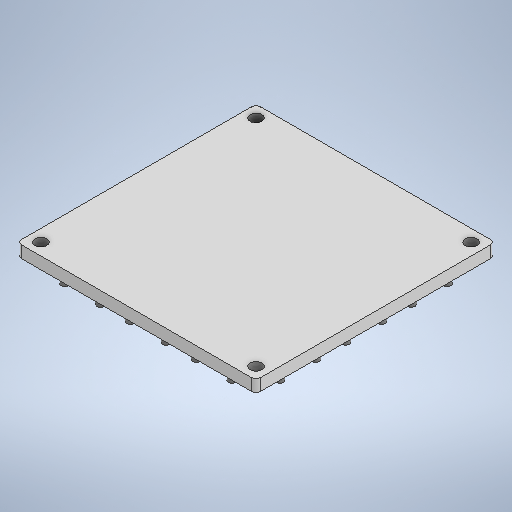
# Autodesk Inventor part: plateau
Saved by Autodesk Inventor 2025 (Build 290162010, 162A)
## iProperties
Created: 2025-02-16
Part Number: plateau
Material: Générique
Document SubType Name: Modeling
Designer: arthu
Density: 1 g/cm^3
Appearance: Par défaut
Author: arthu
Autodesk Inventor part; units mm, degrees
ref_plane "YZ Plane" through (0, 0, 0) normal (1, 0, 0) x (0, 1, 0)
ref_plane "XZ Plane" through (0, 0, 0) normal (0, 1, 0) x (-1, 0, 0)
ref_plane "XY Plane" through (0, 0, 0) normal (0, 0, 1) x (1, 0, 0)
sketch "Esquisse1" plane through (0, 0, 0) normal (0, 1, 0) x (-1, 0, 0)
  line L0 (0, 0) -> (100, 0)
  line L1 (100, 0) -> (100, -100)
  line L2 (100, -100) -> (0, -100)
  line L3 (0, -100) -> (0, 0)
  dimension "d0" = 100
  dimension "d1" = 100
  constraints: 8 end point, 2 parallel, 1 horizontal, 1 perpendicular
  measures "d0" distance of L1.end L2.end
  measures "d1" distance of L0.end L1.end
extrude "Extrusion1" add sketch "Esquisse1" along normal blind 5
sketch "Esquisse3" plane through (0, 0, 0) normal (0, -1, 0) x (1, 0, 0)
  line L0 (0, -100) -> (-100, -100) projected
  line L1 (0, -100) -> (-4.9999, -95)
  circle A0 centre (-4.9999, -95) radius 1.6952
  point P0 (0, 0)
  dimension "d4" = 7.071
  constraints: 2 end point, 1 centre point, 1 coincident
  measures "d4" distance of L0.start L1.end
hole "Perçage1" at (-4.9999, 0, -95) direction (0, 1, 0) diameter 4.9587 depth 5 thread size "M5.5x0.5" class "6H" standard "ISO Metric profile"
pattern_linear "Réseau rectangulaire1" count 2 spacing 90 along (0, 0, 1) count 2 spacing 90 along (-1, 0, 0) of "Perçage1"
fillet "Congé1" radius 2 4 edges at (0, 2.5, 0) (-100, 2.5, 0) (-100, 2.5, -100) (0, 2.5, -100)
sketch "Esquisse7" plane through (0, 0, 0) normal (0, -1, 0) x (1, 0, 0)
  circle A0 centre (-4.9999, -5) radius 2.4794 projected
  circle A1 centre (-94.9999, -95) radius 2.4794 projected
  line L0 (-4.9999, -5) -> (-94.9999, -5)
  line L1 (-94.9999, -5) -> (-94.9999, -95)
  line L2 (-94.9999, -95) -> (-4.9999, -95)
  line L3 (-4.9999, -95) -> (-4.9999, -5)
  line L4 (-49.9999, -5) -> (-49.9999, -95)
  line L5 (-4.9999, -50) -> (-94.9999, -50)
  line L6 (-49.9999, -95) -> (-42.4999, -95)
  line L7 (-49.9999, -95) -> (-57.4999, -95)
  circle A2 centre (-57.4999, -95) radius 1.55
  circle A3 centre (-42.4999, -95) radius 1.55
  line L8 (-94.9999, -95) -> (-84.9999, -95)
  line L9 (-84.9999, -95) -> (-69.9999, -95)
  circle A4 centre (-69.9999, -95) radius 1.55
  circle A5 centre (-84.9999, -95) radius 1.55
  circle A6 centre (-4.9999, -95) radius 2.4794 projected
  line L10 (-4.9999, -95) -> (-14.9999, -95)
  line L11 (-14.9999, -95) -> (-29.9999, -95)
  circle A7 centre (-14.9999, -95) radius 1.55
  circle A8 centre (-29.9999, -95) radius 1.55
  circle A9 centre (-14.9999, -5) radius 1.55
  circle A10 centre (-29.9999, -5) radius 1.55
  circle A11 centre (-42.4999, -5) radius 1.55
  circle A12 centre (-57.4999, -5) radius 1.55
  circle A13 centre (-69.9999, -5) radius 1.55
  circle A14 centre (-84.9999, -5) radius 1.55
  circle A15 centre (-4.9999, -85) radius 1.55
  circle A16 centre (-4.9999, -70) radius 1.55
  circle A17 centre (-4.9999, -57.5) radius 1.55
  circle A18 centre (-4.9999, -42.5) radius 1.55
  circle A19 centre (-4.9999, -30) radius 1.55
  circle A20 centre (-4.9999, -15) radius 1.55
  circle A21 centre (-94.9999, -15) radius 1.55
  circle A22 centre (-94.9999, -30) radius 1.55
  circle A23 centre (-94.9999, -42.5) radius 1.55
  circle A24 centre (-94.9999, -57.5) radius 1.55
  circle A25 centre (-94.9999, -70) radius 1.55
  circle A26 centre (-94.9999, -85) radius 1.55
  point P0 (0, 0)
  dimension "d35" = 7.5
  dimension "d36" = 7.5
  dimension "d37" = 3.1
  dimension "d38" = 3.1
  dimension "d39" = 10
  dimension "d40" = 15
  dimension "d41" = 3.1
  dimension "d42" = 3.1
  dimension "d43" = 10
  dimension "d44" = 15
  dimension "d45" = 3.1
  dimension "d46" = 3.1
  dimension "d49" = 90
  dimension "d56" = 270
  dimension "d60" = 90
  constraints: 24 centre point, 22 end point, 6 coincident, 3 horizontal, 3 midpoint, 1 parallel, 1 perpendicular, 1 vertical, 47 other
  measures "d35" distance of L4.end L6.end
  measures "d36" distance of L4.end L7.end
  measures "d37" diameter of A2
  measures "d38" diameter of A3
  measures "d39" distance of L1.end L8.end
  measures "d40" distance of L8.end L9.end
  measures "d41" diameter of A4
  measures "d42" diameter of A5
  measures "d43" distance of L10.start L10.end
  measures "d44" distance of L10.end L11.end
  measures "d45" diameter of A7
  measures "d46" diameter of A8
  measures "d49" distance of A7.centre A9.centre
  measures "d60" distance of A20.centre A21.centre
extrude "Extrusion3" add sketch "Esquisse7" along normal blind 5 contours A9 L0 | L0 A9 | A20 L3 | L3 A20 | A10 L0 | L0 A10 | A19 L3 | L3 A19 | A11 L0 | L0 A11 | A18 L3 | L3 A18 | A12 L0 | L0 A12 | A17 L3 | L3 A17 | A13 L0 | L0 A13 | A2 L2 | L2 A2 | A3 L2 | L2 A3 | A23 L1 | L1 A23 | A24 L1 | L1 A24 | A16 L3 | L3 A16 | A14 L0 | L0 A14 | A4 L2 | L2 A4 | A8 L2 | L2 A8 | A22 L1 | L1 A22 | A25 L1 | L1 A25 | A15 L3 | L3 A15 | A5 L2 | L2 A5 | A7 L2 | L2 A7 | A21 L1 | L1 A21 | A26 L1 | L1 A26
thread "Filetage1" size "M3.5x0.6" class "6g" standard "ISO Metric profile" full length
thread "Filetage2" size "M3.5x0.6" class "6g" standard "ANSI Metric M Profile" full length
thread "Filetage3" size "M3.5x0.6" class "6g" standard "ANSI Metric M Profile" full length
thread "Filetage4" size "M3.5x0.6" class "6g" standard "ANSI Metric M Profile" full length
thread "Filetage5" size "M3.5x0.6" class "6g" standard "ANSI Metric M Profile" full length
thread "Filetage6" size "M3.5x0.6" class "6g" standard "ANSI Metric M Profile" full length
thread "Filetage7" size "M3.5x0.6" class "6g" standard "ANSI Metric M Profile" full length
thread "Filetage8" size "M3.5x0.6" class "6g" standard "ANSI Metric M Profile" full length
thread "Filetage9" size "M3.5x0.6" class "6g" standard "ANSI Metric M Profile" full length
thread "Filetage10" size "M3.5x0.6" class "6g" standard "ANSI Metric M Profile" full length
thread "Filetage11" size "M3.5x0.6" class "6g" standard "ANSI Metric M Profile" full length
thread "Filetage12" size "M3.5x0.6" class "6g" standard "ANSI Metric M Profile" full length
thread "Filetage13" size "M3.5x0.6" class "6g" standard "ANSI Metric M Profile" full length
thread "Filetage14" size "M3.5x0.6" class "6g" standard "ANSI Metric M Profile" full length
thread "Filetage15" size "M3.5x0.6" class "6g" standard "ANSI Metric M Profile" full length
thread "Filetage16" size "M3.5x0.6" class "6g" standard "ANSI Metric M Profile" full length
thread "Filetage17" size "M3.5x0.6" class "6g" standard "ANSI Metric M Profile" full length
thread "Filetage18" size "M3.5x0.6" class "6g" standard "ANSI Metric M Profile" full length
thread "Filetage19" size "M3.5x0.6" class "6g" standard "ANSI Metric M Profile" full length
thread "Filetage20" size "M3.5x0.6" class "6g" standard "ANSI Metric M Profile" full length
thread "Filetage21" size "M3.5x0.6" class "6g" standard "ANSI Metric M Profile" full length
thread "Filetage22" size "M3.5x0.6" class "6g" standard "ANSI Metric M Profile" full length
thread "Filetage23" size "M3.5x0.6" class "6g" standard "ANSI Metric M Profile" full length
thread "Filetage24" size "M3.5x0.6" class "6g" standard "ANSI Metric M Profile" full length
